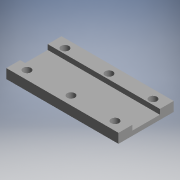
# Autodesk Inventor part: TBCKsupport_plate-MA5150_support_plate
Saved by Autodesk Inventor 2017.3 (Build 213256000, 256)
## iProperties
Part Number: TBCKsupport_plate-MA5150_support_plate
Material: Generic
Catalog Web Link: www.cadenas.de
Description: TBCK_XL, TBCK_L, TBCK_H, TBCK_S3M, TBCK_S5M, TBCK_S8M, TBCK_MA3, TBCK_MA5, TBCK_MA8, TBCK_T5, TBCK_T10, TBCK_AT5, TBCK_AT10_support_plate-Metal Fittings for Timing Belts - Press Prevention Type
Vendor: MISUMI
Document SubType Name: Modeling
Designer: partserver
Manufacturer: MISUMI
Mass: 7.89916 g
Surface Area: 57.8687 cm^2
Volume: 7.89916 cm^3
Density: 1 g/cm^3
Appearance: PSOLRGB-192-192-192
Category: PARTsolutions
Company: MISUMI
Title: TBCKsupport_plate-MA5150_support_plate
Author: Cadenas PARTsolutions
Comments: Metal Fittings for Timing Belts - Press Prevention Type
PSOL_IDENT_0: {$CADENAS_DATA\23d-libs\misumi\metric\48_timing_belts\tbck.prj},351 {VTYP=3D},{NB=TBCKsupport_plate-
PSOL_IDENT_1: MA5150_support_plate},{LINA=TBCKsupport_plate-MA5150_support_plate},{NN=TBCK_XL, TBCK_L, TBCK_H, TBC
PSOL_IDENT_2: K_S3M, TBCK_S5M, TBCK_S8M, TBCK_MA3, TBCK_MA5, TBCK_MA8, TBCK_T5, TBCK_T10, TBCK_AT5, TBCK_AT10_supp
PSOL_IDENT_3: ort_plate},{DATE=30.06.2021 13:24:11},{GEOMDATE=11.02.2010 00:00:00},{VERSION=},{LINEID=120},{WBVAR=
PSOL_IDENT_4: BNW},{WBNUMERIC=}  {NB=TBCKsupport_plate-MA5150_support_plate},{LINA=TBCKsupport_plate-MA5150_suppor
PSOL_IDENT_5: t_plate},{KT=DUMMY},{PN=TBCKsupport_plate-MA5150},{TYPE=TBCK},{MAT=A6N01-T5},{ST=Clear Adonize},{AC=
PSOL_IDENT_6: Hexagon Socket Head Cap Screw},{TB=MA5},{BNW=150},{BNW1='100','100','150','150','250','250'},{W=15.0
PSOL_IDENT_7: },{A=65},{B=32},{T1=6},{T2=5.5},{T3=2.90},{HH=1.70},{L=51},{P=22},{M=M4},{M1=4},{DD=4.5},{AB=M4-10},
PSOL_IDENT_8: {AB1=10},{NMH=6}
NB: TBCKsupport_plate-MA5150_support_plate
NN: TBCK_XL, TBCK_L, TBCK_H, TBCK_S3M, TBCK_S5M, TBCK_S8M, TBCK_MA3, TBCK_MA5, TBCK_MA8, TBCK_T5, TBCK_T10, TBCK_AT5, TBCK_AT10_support_plate
NT: Metal Fittings for Timing Belts - Press Prevention Type
NBSYN: $PN._support_plate
LINA: TBCKsupport_plate-MA5150_support_plate
CATALOG: Misumi
PN: TBCKsupport_plate-MA5150
MAT: A6N01-T5
ST: Clear Adonize
AC: Hexagon Socket Head Cap Screw
TB: MA5
BNW: 150
W: 15
A: 65
B: 32
T1: 6
T2: 5.5
T3: 2.9
HH: 1.7
L: 51
P: 22
M: M4
DD: 4.5
AB: M4-10
NMH: 6
SUPPLIER: MISUMI
ARTICLENO: TBCKsupport_plate-MA5150_support_plate
BOMINFO: TBCKsupport_plate-MA5150_support_plate
CREATOR: CADENAS GmbH
Autodesk Inventor part; units mm, degrees
sketch "Sketch_1" plane through (0, 0, 0) normal (0, 0, 1) x (1, 0, 0)
  line L0 (0, 16) -> (0, -16)
  line L1 (0, -16) -> (65, -16)
  line L2 (65, -16) -> (65, 16)
  line L3 (65, 16) -> (0, 16)
  constraints: 8 end point
extrude "Extrusion1" add sketch "Sketch_1" along normal blind 5.5
sketch "Sketch2" plane through (0, 0, 0) normal (0, 0, -1) x (-1, 0, 0)
  point P0 (-7, 11)
hole "Hole1" at (7, 11, 0) direction (0, 0, 1) diameter 4.5 depth 5.5
pattern_linear "Rectangular Pattern1" count 3 spacing 25.5 along (1, 0, 0) count 2 spacing 22 along (0, -1, 0) of "Hole1"
sketch "Sketch_4" plane through (0, 0, 0) normal (1, 0, 0) x (0, 1, 0)
  line L0 (8, 2.9) -> (-8, 2.9)
  line L1 (-8, 2.9) -> (-8, 0)
  line L2 (-8, 0) -> (8, 0)
  line L3 (8, 0) -> (8, 2.9)
  constraints: 8 end point
extrude "Extrusion2" cut sketch "Sketch_4" along normal blind 65
ref_plane "tbck_XY" through (0, 0, 0) normal (0, 0, 1) x (1, 0, 0)
ref_plane "tbck_YZ" through (0, 0, 0) normal (1, 0, 0) x (0, 1, 0)
ref_plane "tbck_ZX" through (0, 0, 0) normal (0, 1, 0) x (0, 0, 1)
ref_plane "tbck_hole_1_XY" through (7, -11, 5.5) normal (0, 0, 1) x (1, 0, 0)
ref_plane "tbck_hole_1_YZ" through (7, -11, 5.5) normal (1, 0, 0) x (0, 1, 0)
ref_plane "tbck_hole_1_ZX" through (7, -11, 5.5) normal (0, 1, 0) x (0, 0, 1)
ref_plane "tbck_hole_2_XY" through (32.5, -11, 5.5) normal (0, 0, 1) x (1, 0, 0)
ref_plane "tbck_hole_2_YZ" through (32.5, -11, 5.5) normal (1, 0, 0) x (0, 1, 0)
ref_plane "tbck_hole_2_ZX" through (32.5, -11, 5.5) normal (0, 1, 0) x (0, 0, 1)
ref_plane "tbck_hole_3_XY" through (58, -11, 5.5) normal (0, 0, 1) x (1, 0, 0)
ref_plane "tbck_hole_3_YZ" through (58, -11, 5.5) normal (1, 0, 0) x (0, 1, 0)
ref_plane "tbck_hole_3_ZX" through (58, -11, 5.5) normal (0, 1, 0) x (0, 0, 1)
ref_plane "tbck_holes_1_XY" through (7, 11, 5.5) normal (0, 0, 1) x (1, 0, 0)
ref_plane "tbck_holes_1_YZ" through (7, 11, 5.5) normal (1, 0, 0) x (0, 1, 0)
ref_plane "tbck_holes_1_ZX" through (7, 11, 5.5) normal (0, 1, 0) x (0, 0, 1)
ref_plane "tbck_holes_2_XY" through (32.5, 11, 5.5) normal (0, 0, 1) x (1, 0, 0)
ref_plane "tbck_holes_2_YZ" through (32.5, 11, 5.5) normal (1, 0, 0) x (0, 1, 0)
ref_plane "tbck_holes_2_ZX" through (32.5, 11, 5.5) normal (0, 1, 0) x (0, 0, 1)
ref_plane "tbck_holes_3_XY" through (58, 11, 5.5) normal (0, 0, 1) x (1, 0, 0)
ref_plane "tbck_holes_3_YZ" through (58, 11, 5.5) normal (1, 0, 0) x (0, 1, 0)
ref_plane "tbck_holes_3_ZX" through (58, 11, 5.5) normal (0, 1, 0) x (0, 0, 1)
body "Solid1"
